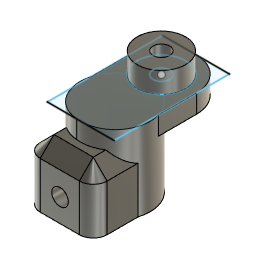
DIYbio orbital shaker - motor coupler (Autodesk Fusion 360 design; units mm, degrees)
Autodesk Fusion 360 part; units mm, degrees
note: some values were not read from the file. Chosen so that the rebuilt part matches the saved one: which sketch regions a step uses; which face or edge a step refers to; which pieces of a blend or face edit are solid.
sketch "Sketch1" plane through (0, 0, 0) normal (0, 0, 1) x (1, 0, 0)
  circle A0 centre (0, 0) radius 2.8
  circle A1 centre (0, 0) radius 7.55
  dimension "d1" = 5.6
  dimension "d2" = 4.75
  constraint coincident A0.centre A1.centre
  measures "d1" diameter of A0
extrude "Extrude1" add sketch "Sketch1" along normal blind 17
ref_plane "WorkPlane1" through (0, -12, 0) normal (0, 1, 0) x (0, 0, 1)
sketch "Sketch3" plane through (0, -12, 0) normal (0, 1, 0) x (1, 0, 0)
  line L0 (-7.3, -13.1) -> (7.2, -13.1)
  line L1 (7.2, -13.1) -> (7.2, 0)
  line L2 (7.2, 0) -> (-7.3, 0)
  line L3 (-7.3, 0) -> (-7.3, -13.1)
  dimension "d15" = 14.5
  dimension "d16" = 13.1
  constraint horizontal L0
  constraint vertical L1
  constraint horizontal L2
  constraint vertical L3
  measures "d15" distance of L0.start L0.end
  measures "d16" distance of L0.start L2.end
extrude "Extrude3" add sketch "Sketch3" along normal up to surface end surface at (7.5406, -0.3763, 11.3333)
sketch "Sketch2" plane through (0, 0, 0) normal (0, 1, 0) x (1, 0, 0)
  circle A0 centre (0, -5) radius 1.8
  dimension "d5" = 3.6
  dimension "d8" = 5
  measures "d5" diameter of A0
  measures "d8" distance of origin A0.centre
extrude "Extrude2" cut sketch "Sketch2" against normal up to surface (12 mm away)
ref_plane "WorkPlane2" through (0, -8, 0) normal (0, 1, 0) x (0, 0, 1)
sketch "Sketch4" plane through (0, -8, 0) normal (0, 1, 0) x (1, 0, 0)
  line L0 (-2.95, -9.6) -> (2.85, -9.6)
  line L1 (2.85, -9.6) -> (2.85, 0)
  line L2 (2.85, 0) -> (-2.95, 0)
  line L3 (-2.95, 0) -> (-2.95, -9.6)
  line L4 (-7.3, 0) -> (-7.3, -13.1)
  line L5 (7.2, -13.1) -> (7.2, 0)
  line L6 (-7.3, -13.1) -> (7.2, -13.1)
  dimension "d21" = 5.8
  dimension "d22" = 9.6
  dimension "d23" = 4.35
  dimension "d24" = 2.6303
  dimension "d25" = 3.5
  constraint horizontal L0
  constraint vertical L1
  constraint horizontal L2
  constraint vertical L3
  measures "d21" distance of L0.start L0.end
  measures "d22" distance of L0.start L2.end
  measures "d23" distance of L3 L4
  measures "d25" distance of L0 L6
extrude "Extrude4" cut sketch "Sketch4" along normal blind 2.5
sketch "Sketch5" plane through (0, 0, 17) normal (0, 0, 1) x (-1, 0, 0)
  circle A0 centre (0, 0) radius 2.8
  circle A1 centre (0, 0) radius 7.55
extrude "Extrude5" add sketch "Sketch5" against normal blind 2 contours A0
sketch "Sketch6" plane through (0, 0, 17) normal (0, 0, 1) x (-1, 0, 0)
  circle A0 centre (0, 0) radius 7.55
  circle A1 centre (0, -10) radius 1.8
  circle A2 centre (0, -10) radius 5.25
  line L0 (7.25, -17.5) -> (-7.25, -17.5)
  line L1 (-7.25, -17.5) -> (-7.25, 7.5)
  line L2 (-7.25, 7.5) -> (7.25, 7.5)
  line L3 (7.25, 7.5) -> (7.25, -17.5)
  dimension "d30" = 3.6
  dimension "d31" = 10
  dimension "d35" = 14.5
  dimension "d36" = 7.25
  dimension "d37" = 7
  dimension "d38" = 25
  dimension "d39" = 7.5
  constraint horizontal L0
  constraint vertical L1
  constraint horizontal L2
  constraint vertical L3
  constraint concentric A1 A2
  measures "d30" diameter of A1
  measures "d31" distance of A0.centre A1.centre
  measures "d35" distance of L1 L3
  measures "d36" distance of A1.centre L3
  measures "d38" distance of L0 L2
  measures "d39" distance of A0.centre L2
extrude "Extrude7" add sketch "Sketch6" against normal blind 4 contours A0 L2 L3 | A0 A2 L0 L1 L3 | A0 A2 picked at (-3.1182, -7.9756)
extrude "Extrude6" add sketch "Sketch6" along normal blind 4.5 contours A0 A2 | A0 A2
fillet "Fillet1" radius 7.1 5 edges at (-7.25, -4.8036, 17) (-4.0587, -7.5, 17) (7.25, 17.5, 15) (-7.25, 17.5, 15) (-7.25, -7.5, 15.05)
fillet "Fillet2" radius 3 2 edges at (7.2, -12, 6.55) (-7.3, -12, 6.55)
chamfer "Chamfer2" distance 3 angle 45 5 edges at (7.2, -5.6361, 13.1) (6.3213, -11.1213, 13.1) (-0.05, -12, 13.1) (-6.4213, -11.1213, 13.1) (-7.3, -5.4634, 13.1)
